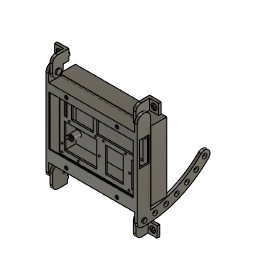
display (Autodesk Fusion 360 design; units mm, degrees)
Autodesk Fusion 360 part; units mm, degrees
note: some values were not read from the file. Set by a fixed rule: which face or edge a step refers to.
sketch "Sketch1" plane through (0, 0, 0) normal (0, 1, 0) x (1, 0, 0) in component "Frame"
  line L0 (0, 0) -> (166, 0)
  line L1 (166, 0) -> (166, -124)
  line L2 (166, -124) -> (0, -124)
  line L3 (0, -124) -> (0, 0)
  circle A0 centre (4.25, -4.25) radius 1.75
  circle A1 centre (161.75, -4.25) radius 1.75
  circle A2 centre (4.25, -119.75) radius 1.75
  circle A3 centre (161.75, -119.75) radius 1.75
  circle A4 centre (17.75, -119.75) radius 1.75
  circle A5 centre (67.45, -119.75) radius 1.75
  circle A6 centre (17.75, -60.75) radius 1.75
  circle A7 centre (67.45, -60.75) radius 1.75
  circle A8 centre (82.45, -60.75) radius 1.75
  circle A9 centre (124.45, -60.75) radius 1.75
  circle A10 centre (131.95, -32.75) radius 1.75
  circle A11 centre (74.95, -32.75) radius 1.75
  line L4 (8.5, -8.5) -> (8.5, -115.5)
  line L5 (157.5, -115.5) -> (157.5, -8.5)
  line L6 (22, -115.5) -> (22, -65)
  line L7 (22, -65) -> (63.2, -65)
  line L8 (63.2, -65) -> (63.2, -115.5)
  line L9 (69.95, -115.5) -> (69.95, -65)
  line L10 (69.95, -56.5) -> (13.5, -56.5)
  line L11 (13.5, -65) -> (13.5, -115.5)
  line L12 (69.95, -65) -> (157.5, -65)
  line L13 (69.95, -56.5) -> (69.95, -8.5)
  line L14 (86.7, -56.5) -> (86.7, -8.5)
  line L15 (120.2, -56.5) -> (120.2, -8.5)
  line L16 (136.2, -56.5) -> (136.2, -8.5)
  line L17 (86.7, -56.5) -> (120.2, -56.5)
  line L18 (136.2, -56.5) -> (157.5, -56.5)
  line L19 (69.95, -8.5) -> (8.5, -8.5)
  line L20 (157.5, -8.5) -> (136.2, -8.5)
  line L21 (120.2, -8.5) -> (86.7, -8.5)
  line L22 (8.5, -115.5) -> (13.5, -115.5)
  line L23 (22, -115.5) -> (63.2, -115.5)
  line L24 (69.95, -115.5) -> (157.5, -115.5)
  circle A12 centre (35, -119.75) radius 1.75
  circle A13 centre (131, -119.75) radius 1.75
  circle A14 centre (131, -4.25) radius 1.75
  circle A15 centre (35, -4.25) radius 1.75
  line L25 (13.5, -65) -> (8.5, -65)
  line L26 (13.5, -56.5) -> (8.5, -56.5)
  circle A16 centre (161.75, -105.5) radius 1.75
  circle A17 centre (161.75, -18.5) radius 1.75
  circle A18 centre (4.25, -18.5) radius 1.75
  circle A19 centre (4.25, -105.5) radius 1.75
  dimension "d1" = 3.5
  dimension "d2" = 2.5
  dimension "d3" = 2.5
  dimension "d4" = 112
  dimension "d5" = 154
  dimension "d6" = 2.5
  dimension "d7" = 2.5
  dimension "d8" = 10
  dimension "d9" = 46.2
  dimension "d10" = 55.5
  dimension "d11" = 7.5
  dimension "d12" = 7.5
  dimension "d13" = 38.5
  dimension "d14" = 28
  dimension "d15" = 2.5
  dimension "d16" = 2.5
  dimension "d17" = 2.5
  dimension "d18" = 2.5
  dimension "d19" = 2.5
  dimension "d20" = 2.5
  dimension "d21" = 2.5
  dimension "d22" = 2.5
  dimension "d23" = 2.5
  dimension "d24" = 2.5
  dimension "d25" = 5
  dimension "d26" = 2.5
  dimension "d27" = 2.5
  dimension "d28" = 2.5
  dimension "d29" = 35
  dimension "d30" = 35
  dimension "d44" = 10
  dimension "d45" = 10
  constraint horizontal L0
  constraint vertical L1
  constraint horizontal L2
  constraint vertical L3
  constraint coincident L0.start L3.end
  constraint equal A0 A1
  constraint equal A0 A2
  constraint equal A0 A3
  constraint vertical A0.centre A2.centre
  constraint horizontal A0.centre A1.centre
  constraint horizontal A2.centre A3.centre
  constraint vertical A1.centre A3.centre
  constraint equal A2 A4
  constraint horizontal A2.centre A4.centre
  constraint horizontal A4.centre A5.centre
  constraint equal A4 A5
  constraint horizontal A6.centre A7.centre
  constraint vertical A5.centre A7.centre
  constraint vertical A4.centre A6.centre
  constraint equal A6 A7
  constraint equal A5 A7
  constraint equal A7 A8
  constraint equal A8 A9
  constraint equal A8 A11
  constraint equal A9 A10
  constraint horizontal A7.centre A8.centre
  constraint horizontal A8.centre A9.centre
  constraint horizontal A10.centre A11.centre
  constraint perpendicular L0 L4
  constraint perpendicular L4 L22
  constraint perpendicular L5 L22
  constraint perpendicular L5 L20
  constraint coincident L6.start L22
  constraint perpendicular L6 L22
  constraint perpendicular L6 L7
  constraint coincident L8.end L22
  constraint perpendicular L8 L22
  constraint coincident L9.start L22
  constraint perpendicular L9 L22
  constraint perpendicular L9 L10
  constraint perpendicular L11 L22
  constraint coincident L5 L12.end
  constraint perpendicular L5 L12
  constraint coincident L5 L18.end
  constraint perpendicular L5 L17
  constraint collinear L7 L12
  constraint coincident L10.start L17
  constraint coincident L13.end L20
  constraint perpendicular L13 L20
  constraint perpendicular L14 L20
  constraint coincident L15.end L20
  constraint perpendicular L15 L20
  constraint coincident L16.start L17
  constraint perpendicular L16 L17
  constraint collinear L9 L13
  constraint collinear L17 L18
  constraint collinear L19 L20
  constraint collinear L20 L21
  constraint collinear L10 L17
  constraint collinear L22 L23
  constraint collinear L23 L24
  constraint horizontal A4.centre A12.centre
  constraint equal A4 A12
  constraint horizontal A3.centre A13.centre
  constraint equal A3 A13
  constraint horizontal A14.centre A15.centre
  constraint equal A0 A15
  constraint equal A14 A15
  constraint vertical A12.centre A15.centre
  constraint vertical A13.centre A14.centre
  constraint horizontal A0.centre A15.centre
  constraint coincident L4 L25.end
  constraint perpendicular L4 L25
  constraint coincident L4 L26.end
  constraint perpendicular L4 L26
  constraint collinear L7 L25
  constraint equal A16 A17
  constraint equal A17 A18
  constraint equal A18 A19
  constraint equal A1 A17
  constraint vertical A16.centre A17.centre
  constraint vertical A1.centre A17.centre
  constraint vertical A0.centre A18.centre
  constraint vertical A18.centre A19.centre
  constraint horizontal A16.centre A19.centre
  constraint horizontal A17.centre A18.centre
  measures "d1" diameter of A0
  measures "d2" distance of L3 A0
  measures "d3" distance of L0 A0
  measures "d4" distance of A0 A2
  measures "d5" distance of A0 A1
  measures "d6" distance of L1 A1
  measures "d7" distance of L2 A2
  measures "d8" distance of A2 A4
  measures "d9" distance of A4 A5
  measures "d10" distance of A4 A6
  measures "d11" horizontal distance of A8.centre A11.centre
  measures "d12" horizontal distance of A9.centre A10.centre
  measures "d13" distance of A8 A9
  measures "d14" vertical distance of A8.centre A11.centre
  measures "d15" distance of A0 L4
  measures "d16" distance of A0 L20
  measures "d17" distance of A2 L22
  measures "d18" distance of A1 L5
  measures "d19" distance of A4 L6
  measures "d20" distance of A4 L11
  measures "d21" distance of A6 L7
  measures "d22" distance of A6 L10
  measures "d23" distance of A5 L8
  measures "d24" distance of A5.centre L9
  measures "d25" distance of A11.centre L13
  measures "d26" distance of A8 L14
  measures "d27" distance of A9 L15
  measures "d28" distance of A10 L16
  measures "d29" distance of L3 A12.centre
  measures "d30" distance of L1 A13.centre
  measures "d44" distance of L20 A17.centre
  measures "d45" distance of L24 A16.centre
extrude "Extrude1" add sketch "Sketch1" along normal blind 3 makes body 1 in component "Frame"
sketch "Sketch4" plane through (0, 0, 0) normal (0, 0, -1) x (1, 0, 0) in component "Frame"
  line L0 (166, 0) -> (0, 0)
  line L1 (0, 0) -> (0, -3)
  line L2 (0, -3) -> (166, -3)
  line L3 (166, -3) -> (166, 0)
  line L4 (157, -3) -> (142, -3)
  line L5 (142, -3) -> (142, -9.5)
  line L6 (157, -9.5) -> (157, -3)
  arc A0 (142, -9.5) -> (157, -9.5) centre (149.5, -9.5) ccw
  circle A1 centre (149.5, -9.5) radius 3.75
  circle A2 centre (149.5, -9.5) radius 5.5
  line L7 (142, -3) -> (136, -3)
  line L8 (136, -3) -> (136, -12.5)
  line L9 (136, -12.5) -> (142, -12.5)
  line L10 (142, -9.5) -> (142, -3)
  line L11 (140.5, -5) -> (137.5, -5)
  line L12 (137.5, -5) -> (137.5, -10.5)
  line L13 (137.5, -10.5) -> (140.5, -10.5)
  line L14 (140.5, -10.5) -> (140.5, -5)
  line L15 (142, -12.5) -> (142.6261, -12.5)
  point P0 (157.5, -3)
  dimension "d34" = 15
  dimension "d35" = 6.5
  dimension "d37" = 0.5
  dimension "d38" = 7.5
  dimension "d39" = 11
  dimension "d46" = 3
  dimension "d47" = 1.5
  dimension "d48" = 1.5
  dimension "d49" = 5.5
  dimension "d50" = 2
  dimension "d51" = 2
  constraint horizontal L4
  constraint vertical L5
  constraint vertical L6
  constraint coincident L2 L4.start
  constraint tangent L5 A0
  constraint equal L5 L6
  constraint concentric A0 A1
  constraint concentric A1 A2
  constraint horizontal L7
  constraint vertical L8
  constraint horizontal L9
  constraint vertical L10
  constraint horizontal L11
  constraint vertical L12
  constraint horizontal L13
  constraint vertical L14
  constraint coincident A0 L15.end
  constraint perpendicular L10 L15
  measures "d34" distance of L5.end L6.start
  measures "d35" distance of L4.start L6.start
  measures "d37" distance of L6 P0
  measures "d38" diameter of A1
  measures "d39" diameter of A2
  measures "d46" distance of L12.end L13.end
  measures "d47" distance of L10 L14
  measures "d48" distance of L8 L12
  measures "d49" distance of L11.end L12.end
  measures "d50" distance of L7 L11
  measures "d51" distance of L9 L13
extrude "Extrude2" add sketch "Sketch4" against normal blind 2.5 separate body contours A2 makes body 2 in component "Frame"
extrude "Extrude3" add sketch "Sketch4" against normal up to surface (8.5 mm away) contours L2 L4 L5 L6 A0 L10 bodies 1 2 in component "Frame"
extrude "Extrude4" add sketch "Sketch4" against normal up to surface (8.5 mm away) contours L2 L5 A0 L7 L8 L9 L10 L15 bodies 1 in component "Frame"
ref_plane "WorkPlane1" through (83, 15, 62) normal (0, 1, 0) x (1, 0, 0) in component "Abdeckung Hinten"
sketch "Sketch1 (2)" plane through (83, 15, 62) normal (0, 1, 0) x (1, 0, 0) in component "Abdeckung Hinten"
  circle A0 centre (78.75, 43.5) radius 1.75
  circle A1 centre (78.75, -43.5) radius 1.75
  circle A2 centre (-78.75, -43.5) radius 1.75
  circle A3 centre (-78.75, 43.5) radius 1.75
  circle A4 centre (-78.75, -43.5) radius 1.75
  circle A5 centre (-78.75, 43.5) radius 1.75
  circle A6 centre (78.75, 43.5) radius 1.75
  circle A7 centre (78.75, -43.5) radius 1.75
  circle A8 centre (78.75, -43.5) radius 3.75
  circle A9 centre (78.75, 43.5) radius 3.75
  circle A10 centre (-78.75, -43.5) radius 3.75
  circle A11 centre (-78.75, 43.5) radius 3.75
  dimension "d56" = 2
  dimension "d57" = 2
  dimension "d58" = 2
  dimension "d59" = 2
  constraint equal A2 A4
  constraint equal A3 A5
  constraint equal A0 A6
  constraint equal A1 A7
  constraint concentric A1 A7
  constraint concentric A0 A6
  constraint concentric A2 A4
  constraint concentric A3 A5
extrude "Extrude1'" add sketch "Sketch1 (2)" along normal blind 2 separate body makes body 3 at (162.7657, 16.3333, 14.8902) makes body 4 at (7.9814, 15.6667, 18.8734) makes body 5 at (162.7657, 16.3333, 101.8902) makes body 6 at (7.884, 16.3333, 104.5747) in component "Abdeckung Hinten"
sketch "Sketch4 (2)" plane through (0, 17, 0) normal (0, 1, 0) x (-1, 0, 0) in component "Abdeckung Hinten"
  circle A0 centre (-4.25, 105.5) radius 1.75
  circle A1 centre (-4.25, 105.5) radius 3.75 construction
  circle A2 centre (-4.25, 105.5) radius 5.75
  circle A3 centre (-4.25, 18.5) radius 5.75
  circle A4 centre (-4.25, 18.5) radius 3.75 construction
  circle A5 centre (-161.75, 18.5) radius 5.75
  circle A6 centre (-161.75, 105.5) radius 5.75
  circle A7 centre (-161.75, 18.5) radius 3.75 construction
  circle A8 centre (-161.75, 105.5) radius 3.75 construction
  circle A9 centre (-4.25, 18.5) radius 1.75
  circle A10 centre (-4.25, 18.5) radius 1.75
  circle A11 centre (-161.75, 18.5) radius 1.75
  circle A12 centre (-161.75, 18.5) radius 1.75
  circle A13 centre (-161.75, 105.5) radius 1.75
  circle A14 centre (-161.75, 105.5) radius 1.75
  dimension "d65" = 2
  constraint concentric A3 A4
  constraint equal A2 A3
  constraint equal A5 A6
  constraint equal A3 A5
  constraint concentric A5 A7
  constraint concentric A6 A8
  constraint concentric A9 A10
  constraint equal A9 A10
  constraint equal A11 A12
  constraint concentric A11 A12
  constraint equal A13 A14
  constraint concentric A13 A14
extrude "Extrude2'" add sketch "Sketch4 (2)" along normal blind 2 bodies 3 4 5 6 in component "Abdeckung Hinten"
sketch "Sketch5" plane through (0, 19, 0) normal (0, 1, 0) x (-1, 0, 0) in component "Abdeckung Hinten"
  circle A0 centre (-4.25, 105.5) radius 1.75
  circle A1 centre (-4.25, 105.5) radius 5.75
  circle A2 centre (-4.25, 105.5) radius 3.35
  circle A3 centre (-4.25, 18.5) radius 3.35
  circle A4 centre (-161.75, 18.5) radius 3.35
  circle A5 centre (-161.75, 105.5) radius 3.35
  circle A6 centre (-161.75, 18.5) radius 1.75
  circle A7 centre (-161.75, 105.5) radius 1.75
  circle A8 centre (-4.25, 18.5) radius 1.75
  circle A9 centre (-161.75, 105.5) radius 5.75
  circle A10 centre (-161.75, 18.5) radius 5.75
  circle A11 centre (-4.25, 18.5) radius 5.75
  circle A12 centre (-4.25, 105.5) radius 5.75
  circle A13 centre (-4.25, 18.5) radius 5.75
  circle A14 centre (-161.75, 18.5) radius 5.75
  circle A15 centre (-161.75, 105.5) radius 5.75
  dimension "d68" = 1.6
  dimension "d69" = 1.4
  constraint equal A2 A3
  constraint equal A3 A4
  constraint equal A4 A5
  constraint concentric A4 A6
  constraint concentric A5 A7
  constraint concentric A3 A8
  constraint concentric A7 A9
  constraint concentric A4 A10
  constraint concentric A8 A11
  constraint concentric A0 A12
  constraint equal A1 A12
  constraint equal A11 A13
  constraint equal A10 A14
  constraint equal A9 A15
extrude "Extrude3'" add sketch "Sketch5" along normal blind 12 contours A1 A12 | A9 A15 | A10 A14 | A11 A13 bodies 3 4 5 6 in component "Abdeckung Hinten"
ref_plane "WorkPlane2" through (161.75, 31, 105.5) normal (0, 1, 0) x (-1, 0, 0) in component "Abdeckung Hinten"
sketch "Sketch8" plane through (161.75, 31, 105.5) normal (0, 1, 0) x (1, 0, 0) in component "Abdeckung Hinten"
  line L0 (7.75, -22) -> (-165.25, -22)
  line L1 (-165.25, -22) -> (-165.25, 109)
  line L2 (-165.25, 109) -> (7.75, 109)
  line L3 (7.75, 109) -> (7.75, -22)
  line L4 (4.25, 105.5) -> (4.25, -18.5)
  line L5 (4.25, -18.5) -> (-161.75, -18.5)
  line L6 (-161.75, 105.5) -> (4.25, 105.5)
  line L7 (-161.75, -18.5) -> (-161.75, 105.5)
  circle A0 centre (-157.5, 0) radius 3.35
  circle A1 centre (-157.5, 0) radius 3.35
  circle A2 centre (-157.5, 87) radius 3.35
  circle A3 centre (-157.5, 87) radius 3.35
  circle A4 centre (0, 87) radius 3.35
  circle A5 centre (0, 87) radius 3.35
  circle A6 centre (0, 0) radius 3.35
  circle A7 centre (0, 0) radius 3.35
  dimension "d81" = 3.5
  dimension "d82" = 3.5
  dimension "d83" = 3.5
  dimension "d84" = 3.5
  constraint horizontal L0
  constraint vertical L1
  constraint horizontal L2
  constraint vertical L3
  constraint equal A0 A1
  constraint concentric A0 A1
  constraint equal A2 A3
  constraint concentric A2 A3
  constraint equal A4 A5
  constraint concentric A4 A5
  constraint equal A6 A7
  constraint concentric A6 A7
  measures "d81" distance of L3 L4
  measures "d82" distance of L0 L5
  measures "d83" distance of L2 L6
  measures "d84" distance of L1 L7
extrude "Extrude4'" add sketch "Sketch8" along normal blind 2 contours L0 L1 L2 L3 | L4 L5 L6 L7 bodies 3 4 5 6 in component "Abdeckung Hinten"
sketch "Sketch9" plane through (0, 31, 0) normal (0, -1, 0) x (1, 0, 0) in component "Abdeckung Hinten"
  circle A0 centre (4.25, 105.5) radius 5.75
  circle A1 centre (161.75, 105.5) radius 5.75
  circle A2 centre (4.25, 18.5) radius 5.75
  line L0 (-3.5, -3.5) -> (169.5, -3.5)
  line L1 (169.5, -3.5) -> (169.5, 127.5)
  line L2 (169.5, 127.5) -> (-3.5, 127.5)
  line L3 (-3.5, 127.5) -> (-3.5, -3.5)
  circle A3 centre (161.75, 18.5) radius 5.75
  line L4 (-0.5, -0.5) -> (166.5, -0.5)
  line L5 (166.5, -0.5) -> (166.5, 124.5)
  line L6 (166.5, 124.5) -> (-0.5, 124.5)
  line L7 (-0.5, 124.5) -> (-0.5, -0.5)
  dimension "d87" = -3
extrude "Extrude5" add sketch "Sketch9" along normal up to surface (31 mm away) bodies 3 in component "Abdeckung Hinten"
sketch "Sketch10" plane through (0, 0, 0) normal (0, -1, 0) x (1, 0, 0) in component "Abdeckung Hinten"
  arc A0 (-0.5, 108.7404) -> (-0.5, 102.2596) centre (4.25, 105.5) ccw
  line L0 (-0.5, 108.7404) -> (-0.5, 124.5)
  line L1 (-0.5, 124.5) -> (166.5, 124.5)
  line L2 (166.5, 124.5) -> (166.5, 108.7404)
  arc A1 (166.5, 102.2596) -> (166.5, 108.7404) centre (161.75, 105.5) ccw
  line L3 (166.5, 102.2596) -> (166.5, 21.7404)
  arc A2 (166.5, 15.2596) -> (166.5, 21.7404) centre (161.75, 18.5) ccw
  line L4 (166.5, 15.2596) -> (166.5, -0.5)
  line L5 (166.5, -0.5) -> (-0.5, -0.5)
  line L6 (-0.5, -0.5) -> (-0.5, 15.2596)
  arc A3 (-0.5, 21.7404) -> (-0.5, 15.2596) centre (4.25, 18.5) ccw
  line L7 (-0.5, 21.7404) -> (-0.5, 102.2596)
  line L8 (169.5, 127.5) -> (-3.5, 127.5)
  line L9 (-3.5, 127.5) -> (-3.5, -3.5)
  line L10 (-3.5, -3.5) -> (169.5, -3.5)
  line L11 (169.5, -3.5) -> (169.5, 127.5)
  line L12 (-1.9, -1.9) -> (167.9, -1.9)
  line L13 (167.9, -1.9) -> (167.9, 125.9)
  line L14 (167.9, 125.9) -> (-1.9, 125.9)
  line L15 (-1.9, 125.9) -> (-1.9, -1.9)
  dimension "d90" = -1.6
extrude "Extrude6" cut sketch "Sketch10" against normal blind 3 contours L8 L9 L10 L11 bodies 3 in component "Abdeckung Hinten"
sketch "Sketch11" plane through (0, 0, -0.5) normal (0, 0, 1) x (-1, 0, 0) in component "Abdeckung Hinten"
  line L0 (0.5, 0) -> (-166.5, 0)
  line L1 (-166.5, 0) -> (-166.5, -31)
  line L2 (-166.5, -31) -> (0.5, -31)
  line L3 (0.5, -31) -> (0.5, 0)
  line L4 (-157, -3) -> (-136, -3) construction
  line L5 (-157, -9.5) -> (-157, -3) construction
  line L6 (0, -3) -> (-166, -3)
  line L7 (-157, -9.5) -> (-157, -3)
  line L8 (-136, -3) -> (-136, -12.5) construction
  line L9 (-136, -3) -> (-136, -12.5)
  arc A0 (-157, -9.5) -> (-142.6261, -12.5) centre (-149.5, -9.5) ccw
  arc A1 (-157, -9.5) -> (-142.6261, -12.5) centre (-149.5, -9.5) ccw construction
  line L10 (-142.6261, -12.5) -> (-136, -12.5) construction
  line L11 (-137, -4) -> (-137, -11.5)
  line L12 (-143.3153, -11.5) -> (-137, -11.5)
  arc A2 (-156, -9.5) -> (-143.3153, -11.5) centre (-149.5, -9.5) ccw
  line L13 (-156, -9.5) -> (-156, -4)
  line L14 (-156, -4) -> (-137, -4)
  dimension "d93" = -1
  constraint horizontal L4
  constraint vertical L5
  constraint collinear L4 L6
  constraint collinear L5 L7
  constraint perpendicular L6 L8
  constraint equal L8 L9
  constraint collinear L8 L9
  constraint equal A0 A1
  constraint concentric A0 A1
  constraint coincident A0.end A1.end
extrude "Extrude7" cut sketch "Sketch11" against normal up to surface (3 mm away) contours L11 L12 A2 L13 L14 bodies 3 in component "Abdeckung Hinten"
ref_plane "WorkPlane1" through (83, -12, 62) normal (0, -1, 0) x (-1, 0, 0) in component "Display Halterung"
sketch "Sketch1 (3)" plane through (83, -12, 62) normal (0, -1, 0) x (1, 0, 0) in component "Display Halterung"
  circle A0 centre (-48, 57.75) radius 1.75
  circle A1 centre (48, 57.75) radius 1.75
  circle A2 centre (-48, -57.75) radius 1.75
  circle A3 centre (48, -57.75) radius 1.75
  circle A4 centre (-48, 57.75) radius 1.75
  circle A5 centre (48, 57.75) radius 1.75
  circle A6 centre (48, -57.75) radius 1.75
  circle A7 centre (-48, -57.75) radius 1.75
  circle A8 centre (-48, 57.75) radius 3.75
  circle A9 centre (48, 57.75) radius 3.75
  circle A10 centre (48, -57.75) radius 3.75
  circle A11 centre (-48, -57.75) radius 3.75
  dimension "d97" = 2
  dimension "d98" = 2
  dimension "d99" = 2
  dimension "d100" = 2
  constraint equal A0 A4
  constraint equal A1 A5
  constraint equal A3 A6
  constraint equal A2 A7
  constraint concentric A2 A7
  constraint concentric A3 A6
  constraint concentric A1 A5
  constraint concentric A0 A4
extrude "Extrude1''" add sketch "Sketch1 (3)" along normal blind 6.5 separate body makes body 7 at (132.0157, -16.3333, 7.8598) makes body 8 at (132.0157, -16.3333, 123.3598) makes body 9 at (38.7314, -14.1667, 3.8766) makes body 10 at (38.634, -16.3333, 120.6753) in component "Display Halterung"
ref_plane "WorkPlane2" through (83, -18.5, 62) normal (0, -1, 0) x (-1, 0, 0) in component "Display Halterung"
sketch "Sketch2" plane through (83, -18.5, 62) normal (0, -1, 0) x (1, 0, 0) in component "Display Halterung"
  line L0 (-86.5, 65.5) -> (86.5, 65.5)
  line L1 (86.5, 65.5) -> (86.5, -65.5)
  line L2 (86.5, -65.5) -> (-86.5, -65.5)
  line L3 (-86.5, -65.5) -> (-86.5, 65.5)
  line L4 (-86.5, 65.5) -> (86.5, 65.5)
  line L5 (86.5, 65.5) -> (86.5, -65.5)
  line L6 (86.5, -65.5) -> (-86.5, -65.5)
  line L7 (-86.5, -65.5) -> (-86.5, 65.5)
  line L8 (-83, 53.5) -> (83, 53.5)
  line L9 (83, 53.5) -> (83, -47.6)
  line L10 (83, -47.6) -> (-83, -47.6)
  line L11 (-83, -47.6) -> (-83, 53.5)
  line L12 (-83, 62) -> (-83, -62)
  line L13 (83, -62) -> (83, 62)
  line L14 (74.5, 53.5) -> (-13.05, 53.5)
  circle A0 centre (48, -57.75) radius 1.75
  circle A1 centre (-48, 57.75) radius 1.75
  circle A2 centre (48, 57.75) radius 1.75
  circle A3 centre (-48, -57.75) radius 1.75
  dimension "d105" = 166
  dimension "d106" = 100.8
  dimension "d107" = 8.4
  dimension "d108" = 3.5
  dimension "d109" = 3.5
  dimension "d110" = 3.5
  constraint horizontal L0
  constraint vertical L1
  constraint horizontal L2
  constraint vertical L3
  constraint collinear L0 L4
  constraint collinear L1 L5
  constraint collinear L2 L6
  constraint collinear L3 L7
  constraint horizontal L8
  constraint vertical L9
  constraint horizontal L10
  constraint vertical L11
  constraint collinear L11 L12
  constraint collinear L9 L13
  constraint collinear L8 L14
  measures "d105" distance of L8.start L8.end
  measures "d107" distance of L10 A0
  measures "d108" diameter of A1
  measures "d109" diameter of A2
  measures "d110" diameter of A3
extrude "Extrude2''" add sketch "Sketch2" along normal blind 2.8 bodies 7 8 9 10 in component "Display Halterung"
sketch "Sketch3" plane through (0, -21.3, 0) normal (0, -1, 0) x (1, 0, 0) in component "Display Halterung"
  circle A0 centre (131, 119.75) radius 1.75
  circle A1 centre (35, 119.75) radius 1.75
  circle A2 centre (131, 4.25) radius 1.75
  line L0 (166, 115.5) -> (166, 14.4) construction
  line L1 (166, 14.4) -> (0, 14.4) construction
  line L2 (0, 14.4) -> (0, 115.5) construction
  line L3 (0, 115.5) -> (166, 115.5) construction
  circle A3 centre (35, 4.25) radius 1.75
  line L4 (-3.5, -3.5) -> (169.5, -3.5)
  line L5 (169.5, -3.5) -> (169.5, 127.5)
  line L6 (169.5, 127.5) -> (-3.5, 127.5)
  line L7 (-3.5, 127.5) -> (-3.5, -3.5)
  line L8 (2, 112.5) -> (162, 112.5)
  line L9 (162, 112.5) -> (162, 18.9)
  line L10 (162, 18.9) -> (2, 18.9)
  line L11 (2, 18.9) -> (2, 112.5)
  dimension "d113" = 4
  dimension "d114" = 3
  dimension "d115" = 2
  dimension "d116" = 4.5
  constraint horizontal L8
  constraint vertical L9
  constraint horizontal L10
  constraint vertical L11
  measures "d113" distance of L0 L9
  measures "d114" distance of L3 L8
  measures "d115" distance of L2 L11
  measures "d116" distance of L1 L10
extrude "Extrude3''" add sketch "Sketch3" along normal blind 1.5 bodies 7 in component "Display Halterung"
sketch "Sketch4 (3)" plane through (0, -22.8, 0) normal (0, -1, 0) x (1, 0, 0) in component "Display Halterung"
  circle A0 centre (35, 119.75) radius 1.75
  circle A1 centre (131, 4.25) radius 1.75
  circle A2 centre (35, 4.25) radius 1.75
  circle A3 centre (131, 119.75) radius 1.75
  line L0 (162, 18.9) -> (2, 18.9)
  line L1 (2, 18.9) -> (2, 112.5)
  line L2 (2, 112.5) -> (162, 112.5)
  line L3 (162, 112.5) -> (162, 18.9)
  line L4 (-3.5, 127.5) -> (-3.5, -3.5)
  line L5 (-3.5, -3.5) -> (169.5, -3.5)
  line L6 (169.5, -3.5) -> (169.5, 127.5)
  line L7 (169.5, 127.5) -> (-3.5, 127.5)
  circle A4 centre (131, 119.75) radius 3.25
  circle A5 centre (35, 119.75) radius 3.25
  circle A6 centre (131, 4.25) radius 3.25
  circle A7 centre (35, 4.25) radius 3.25
  dimension "d119" = 1.5
  dimension "d120" = 1.5
  dimension "d121" = 1.5
  dimension "d122" = 1.5
extrude "Extrude4''" cut sketch "Sketch4 (3)" against normal blind 2 contours A4 | A5 | A6 | A7 bodies 7 in component "Display Halterung"
sketch "Sketch5 (2)" plane through (0, -18.5, 0) normal (0, 1, 0) x (-1, 0, 0) in component "Display Halterung"
  circle A0 centre (-35, 119.75) radius 3.75
  circle A1 centre (-35, 4.25) radius 3.75
  circle A2 centre (-131, 119.75) radius 3.75
  line L0 (-169.5, -3.5) -> (3.5, -3.5)
  line L1 (3.5, -3.5) -> (3.5, 127.5)
  line L2 (3.5, 127.5) -> (-169.5, 127.5)
  line L3 (-169.5, 127.5) -> (-169.5, -3.5)
  line L4 (-166, 14.4) -> (-166, 115.5)
  line L5 (-166, 115.5) -> (0, 115.5)
  line L6 (0, 115.5) -> (0, 14.4)
  line L7 (0, 14.4) -> (-166, 14.4)
  circle A3 centre (-131, 4.25) radius 3.75
  line L8 (-166.5, 124.5) -> (0.5, 124.5)
  line L9 (0.5, 124.5) -> (0.5, -0.5)
  line L10 (0.5, -0.5) -> (-166.5, -0.5)
  line L11 (-166.5, -0.5) -> (-166.5, 124.5)
  line L12 (0.5, 124.5) -> (0.5, -0.5)
  line L13 (-166.5, 124.5) -> (0.5, 124.5)
  line L14 (-166.5, -0.5) -> (-166.5, 124.5)
  line L15 (0.5, -0.5) -> (-166.5, -0.5)
  constraint horizontal L8
  constraint vertical L9
  constraint horizontal L10
  constraint vertical L11
  constraint collinear L9 L12
  constraint collinear L8 L13
  constraint collinear L11 L14
  constraint collinear L10 L15
extrude "Extrude5'" add sketch "Sketch5 (2)" along normal up to surface (18.2 mm away) contours L0 L1 L2 L3 bodies 7 in component "Display Halterung"
sketch "Sketch6" plane through (0, -0.3, 0) normal (0, 1, 0) x (-1, 0, 0) in component "Display Halterung"
  line L0 (-166.5, 124.5) -> (0.5, 124.5)
  line L1 (0.5, 124.5) -> (0.5, -0.5)
  line L2 (0.5, -0.5) -> (-166.5, -0.5)
  line L3 (-166.5, -0.5) -> (-166.5, 124.5)
  line L4 (3.5, 127.5) -> (-169.5, 127.5)
  line L5 (-169.5, 127.5) -> (-169.5, -3.5)
  line L6 (-169.5, -3.5) -> (3.5, -3.5)
  line L7 (3.5, -3.5) -> (3.5, 127.5)
  line L8 (-168.2, 126.2) -> (2.2, 126.2)
  line L9 (2.2, 126.2) -> (2.2, -2.2)
  line L10 (2.2, -2.2) -> (-168.2, -2.2)
  line L11 (-168.2, -2.2) -> (-168.2, 126.2)
  line L12 (1.9, 125.9) -> (1.9, -1.9)
  line L13 (-167.9, 125.9) -> (1.9, 125.9)
  line L14 (-167.9, -1.9) -> (-167.9, 125.9)
  line L15 (1.9, -1.9) -> (-167.9, -1.9)
  dimension "d127" = 0.3
  dimension "d128" = 0.3
  dimension "d129" = 0.3
  dimension "d130" = 0.3
  constraint horizontal L8
  constraint vertical L9
  constraint horizontal L10
  constraint vertical L11
  measures "d127" distance of L9 L12
  measures "d128" distance of L8 L13
  measures "d129" distance of L11 L14
  measures "d130" distance of L10 L15
extrude "Extrude6'" add sketch "Sketch6" along normal up to surface (2.8 mm away) contours L4 L5 L6 L7 bodies 7 in component "Display Halterung"
sketch "Sketch7" plane through (166.5, 0, 0) normal (-1, 0, 0) x (0, -1, 0) in component "Display Halterung"
  line L0 (0.3, 124.5) -> (0.3, -0.5)
  line L1 (0.3, -0.5) -> (18.5, -0.5)
  line L2 (18.5, -0.5) -> (18.5, 124.5)
  line L3 (18.5, 124.5) -> (0.3, 124.5)
  line L4 (0.3, 115) -> (19.3, 115)
  line L5 (19.3, 115) -> (19.3, 68)
  line L6 (19.3, 68) -> (0.3, 68)
  line L7 (0.3, 68) -> (0.3, 115)
  line L8 (0, 124) -> (-3, 124)
  dimension "d133" = 19
  dimension "d134" = 9
  dimension "d135" = 47
  constraint horizontal L4
  constraint vertical L5
  constraint horizontal L6
  constraint vertical L7
  constraint coincident L0 L4.start
  measures "d133" distance of L4.start L4.end
  measures "d134" distance of L4 L8
  measures "d135" distance of L4.start L6.end
extrude "Extrude7'" cut sketch "Sketch7" against normal up to surface (3 mm away) contours L0 L2 L4 L6 L7 bodies 7 in component "Display Halterung"
sketch "Sketch9 (2)" plane through (-3.5, 0, 0) normal (-1, 0, 0) x (0, -1, 0) in component "Display Halterung"
  line L0 (-2.5, -3.5) -> (22.8, -3.5)
  line L1 (22.8, -3.5) -> (22.8, 127.5)
  line L2 (22.8, 127.5) -> (-2.5, 127.5)
  line L3 (-2.5, 127.5) -> (-2.5, -3.5)
  line L4 (-2.5, 127.5) -> (22.8, 127.5)
  line L5 (22.8, 127.5) -> (22.8, 142.5)
  line L6 (-2.5, 142.5) -> (-2.5, 127.5)
  arc A0 (22.8, 142.5) -> (-2.5, 142.5) centre (10.15, 142.5) ccw
  dimension "d140" = 15
  dimension "d141" = 25.3
  constraint horizontal L4
  constraint vertical L5
  constraint vertical L6
  constraint coincident L2.end L3.start
  constraint tangent L5 A0
  constraint collinear L1 L5
  constraint tangent L6 A0
  measures "d140" distance of L2.end L6.start
  measures "d141" distance of L5.end L6.start
extrude "Extrude8" add sketch "Sketch9 (2)" against normal blind 5 contours L2 L4 L5 L6 A0 bodies 7 in component "Display Halterung"
extrude "Extrude9" add sketch "Sketch9 (2)" along normal blind 5 from surface at -173 contours L2 L4 L5 L6 A0 bodies 7 in component "Display Halterung"
sketch "Sketch10 (2)" plane through (1.5, 0, 0) normal (1, 0, 0) x (0, 1, 0) in component "Display Halterung"
  arc A0 (2.5, 142.5) -> (-22.8, 142.5) centre (-10.15, 142.5) ccw
  line L0 (-22.8, 142.5) -> (-22.8, 127.5)
  line L1 (-22.8, 127.5) -> (2.5, 127.5)
  line L2 (2.5, 127.5) -> (2.5, 142.5)
  circle A1 centre (-10.15, 142.5) radius 5
  dimension "d147" = 10
  constraint concentric A0 A1
  measures "d147" diameter of A1
extrude "Extrude10" add sketch "Sketch10 (2)" along normal blind 7 contours A1 bodies 7 in component "Display Halterung"
extrude "Extrude11" add sketch "Sketch10 (2)" against normal blind 7 from surface at 163 contours A1 bodies 7 in component "Display Halterung"
sketch "Sketch11 (2)" plane through (-3.5, 0, 0) normal (-1, 0, 0) x (0, -1, 0) in component "Display Halterung"
  circle A0 centre (10.15, 142.5) radius 5
  arc A1 (-98.0373, 34.3127) -> (10.15, -10.5) centre (10.15, 142.5) ccw
  line L0 (10.15, 142.5) -> (-98.0373, 34.3127) construction
  line L1 (10.15, 142.5) -> (10.15, -10.5) construction
  arc A2 (-112.1795, 20.1705) -> (10.15, -30.5) centre (10.15, 142.5) ccw
  line L2 (22.8, -3.5) -> (-2.5, -3.5)
  line L3 (-2.5, -3.5) -> (-2.5, -9.9762)
  line L4 (22.8, -20.5) -> (22.8, -3.5)
  line L5 (-2.5, -3.5) -> (22.8, -3.5)
  line L6 (-2.5, 142.5) -> (-2.5, -3.5)
  line L7 (22.8, -3.5) -> (22.8, 142.5)
  line L8 (10.15, -30.5) -> (12.8, -30.5)
  arc A3 (-98.0373, 34.3127) -> (-112.1795, 20.1705) centre (-105.1084, 27.2416) ccw
  circle A4 centre (10.15, -20.5) radius 4.4
  circle A5 centre (-11.1258, -19.1055) radius 4.4
  circle A6 centre (-32.0375, -14.9459) radius 4.4
  circle A7 centre (-52.2274, -8.0924) radius 4.4
  circle A8 centre (-71.35, 1.3379) radius 4.4
  circle A9 centre (-89.0781, 13.1834) radius 4.4
  circle A10 centre (-105.1084, 27.2416) radius 4.4
  arc A11 (12.8, -30.5) -> (22.8, -20.5) centre (12.8, -20.5) ccw
  point P0 (22.8, -30.5)
  dimension "d182" = 45
  dimension "d183" = 20
  dimension "d184" = 27
  dimension "d199" = 8.8
  dimension "d200" = 12.65
  dimension "d201" = 25.3
  dimension "d202" = 10
  dimension "d204" = -45
  dimension "d205" = 10
  constraint coincident A0.centre A1.centre
  constraint horizontal L2
  constraint vertical L3
  constraint vertical L4
  constraint collinear L2 L5
  constraint collinear L3 L6
  constraint collinear L4 L7
  constraint perpendicular L4 L8
  constraint tangent A2 L8
  constraint coincident A1 L3.end
  constraint tangent A1 A3
  constraint coincident P0 L4
  constraint coincident P0 L8
  constraint tangent L4 A11
  constraint tangent L8 A11
  measures "d182" angle of L0 L1
  measures "d184" distance of L2.start P0
  measures "d199" diameter of A4
  measures "d200" distance of L4 A4.centre
  measures "d201" distance of L2.start L2.end
  measures "d202" distance of L8 A4.centre
  measures "d205" radius of A11
extrude "Extrude18" add sketch "Sketch11 (2)" against normal up to surface (5 mm away) contours A1 A2 L2 L3 L4 L5 L8 A3 A11 bodies 7 in component "Display Halterung"
extrude "Extrude19" add sketch "Sketch11 (2)" along normal up to surface (5 mm away) from surface at -173 contours A1 A2 L2 L3 L4 L5 L8 A3 A11 bodies 7 in component "Display Halterung"
sketch "Sketch1 (4)" plane through (1.5, 0, 0) normal (1, 0, 0) x (0, 1, 0) in component "Geruesthalterung Top"
  circle A0 centre (-10.15, 142.5) radius 5
  arc A1 (2.5, 142.5) -> (-22.8, 142.5) centre (-10.15, 142.5) ccw construction
  line L0 (-22.8, 142.5) -> (-22.8, 127.5)
  line L1 (-22.8, 127.5) -> (2.5, 127.5)
  line L2 (2.5, 127.5) -> (2.5, 142.5)
  circle A2 centre (-10.15, 142.5) radius 5.25
  line L3 (-0.15, 142.5) -> (-0.15, 149.5)
  line L4 (10.5, 169.5) -> (-10.15, 169.5)
  line L5 (-20.15, 159.5) -> (-20.15, 142.5)
  arc A3 (-20.15, 142.5) -> (-0.15, 142.5) centre (-10.15, 142.5) ccw
  arc A4 (-10.15, 169.5) -> (-20.15, 159.5) centre (-10.15, 159.5) ccw
  line L6 (10.5, 169.5) -> (10.5, 149.5)
  line L7 (10.5, 149.5) -> (-0.15, 149.5)
  dimension "d206" = 10.5
  dimension "d208" = 20
  dimension "d230" = 10
  dimension "d273" = 8
  dimension "d274" = 20
  dimension "d275" = 7
  constraint concentric A0 A2
  constraint concentric A0 A3
  constraint vertical L3
  constraint vertical L5
  constraint tangent L5 A3
  constraint tangent L3 A3
  constraint vertical L6
  constraint horizontal L7
  constraint tangent L5 A4
  constraint tangent L4 A4
  constraint horizontal L4
  measures "d206" diameter of A2
  measures "d208" diameter of A3
  measures "d230" radius of A4
  measures "d273" distance of L2 L6
  measures "d274" distance of L4.start L6.end
  measures "d275" distance of L3.start L3.end
extrude "Extrude1'''" add sketch "Sketch1 (4)" along normal blind 5 separate body contours L3 L4 L5 A3 A4 L6 L7 makes body 11 in component "Geruesthalterung Top"
sketch "Sketch2 (2)" plane through (1.5, 0, 0) normal (-1, 0, 0) x (0, -1, 0) in component "Geruesthalterung Top"
  circle A0 centre (10.15, 142.5) radius 5.25
  arc A1 (0.15, 142.5) -> (20.15, 142.5) centre (10.15, 142.5) ccw
  line L0 (20.15, 142.5) -> (20.15, 159.5)
  line L1 (10.15, 169.5) -> (-10.5, 169.5)
  line L2 (0.15, 149.5) -> (0.15, 142.5)
  line L3 (-10.5, 169.5) -> (-5.5, 169.5)
  line L4 (-5.5, 169.5) -> (-5.5, 149.5)
  line L5 (-5.5, 149.5) -> (-10.5, 149.5)
  line L6 (-10.5, 149.5) -> (-10.5, 169.5)
  arc A2 (20.15, 159.5) -> (10.15, 169.5) centre (10.15, 159.5) ccw
  line L7 (-10.5, 169.5) -> (-10.5, 149.5)
  line L8 (-10.5, 149.5) -> (0.15, 149.5)
  dimension "d212" = 20
  dimension "d213" = 5
  constraint horizontal L3
  constraint vertical L4
  constraint horizontal L5
  constraint vertical L6
  constraint coincident L1.end L3.start
  measures "d212" distance of L1.end L5.end
  measures "d213" distance of L1.end L3.end
extrude "Extrude2'''" add sketch "Sketch2 (2)" along normal blind 17 contours L1 L3 L4 L5 L6 L7 L8 bodies 11 in component "Geruesthalterung Top"
extrude "Extrude3'''" add sketch "Sketch1 (4)" against normal blind 5 from surface at 163 separate body contours L3 L4 L5 A3 A4 L6 L7 makes body 12 in component "Geruesthalterung Top"
extrude "Extrude4'''" add sketch "Sketch2 (2)" against normal blind 17 from surface at -163 contours L1 L3 L4 L5 L6 L7 L8 bodies 12 in component "Geruesthalterung Top"
sketch "Sketch3 (2)" plane through (0, 5.5, 0) normal (0, -1, 0) x (1, 0, 0) in component "Geruesthalterung Top"
  line L0 (1.5, 149.5) -> (1.5, 169.5)
  line L1 (1.5, 169.5) -> (-15.5, 169.5)
  line L2 (-15.5, 169.5) -> (-15.5, 149.5)
  line L3 (-15.5, 149.5) -> (1.5, 149.5)
  line L4 (1.5, 159.5) -> (-15.5, 159.5) construction
  line L5 (-7, 169.5) -> (-7, 149.5) construction
  circle A0 centre (-7, 159.5) radius 5.5
  circle A1 centre (-7, 159.5) radius 2.75
  dimension "d222" = 11
  dimension "d223" = 5.5
  constraint midpoint L0 L4.start
  constraint midpoint L2 L4.end
  constraint midpoint L1 L5.start
  constraint midpoint L3 L5.end
  constraint midpoint L5 A0.centre
  constraint concentric A0 A1
  measures "d222" diameter of A0
  measures "d223" diameter of A1
sketch "Sketch4 (4)" plane through (0, 5.5, 0) normal (0, -1, 0) x (1, 0, 0) in component "Geruesthalterung Top"
  line L0 (164.5, 169.5) -> (164.5, 149.5)
  line L1 (164.5, 149.5) -> (181.5, 149.5)
  line L2 (181.5, 149.5) -> (181.5, 169.5)
  line L3 (181.5, 169.5) -> (164.5, 169.5)
  line L4 (173, 169.5) -> (173, 149.5) construction
  line L5 (181.5, 159.5) -> (164.5, 159.5) construction
  circle A0 centre (173, 159.5) radius 5.5
  circle A1 centre (173, 159.5) radius 2.75
  dimension "d224" = 11
  dimension "d225" = 5.5
  constraint midpoint L3 L4.start
  constraint midpoint L1 L4.end
  constraint midpoint L2 L5.start
  constraint midpoint L0 L5.end
  constraint midpoint L5 A0.centre
  constraint concentric A0 A1
  measures "d224" diameter of A0
  measures "d225" diameter of A1
extrude "Extrude5''" cut sketch "Sketch4 (4)" sketch "Sketch3 (2)" along normal up to surface contours A1 of sketch 2 contours A1 end surface through (164.5, 10.5, 169.5) normal (0, 1, 0) offset 0 bodies 11 12 in component "Geruesthalterung Top"
extrude "Extrude6''" cut sketch "Sketch4 (4)" sketch "Sketch3 (2)" against normal blind 2 contours A0 of sketch 2 contours A0 bodies 11 12 in component "Geruesthalterung Top"
sketch "Sketch5 (3)" plane through (0, 10.5, 0) normal (0, 1, 0) x (-1, 0, 0) in component "Geruesthalterung Top"
  circle A0 centre (7, 159.5) radius 2.75
  line L0 (-6.5, 149.5) -> (15.5, 149.5)
  line L1 (15.5, 149.5) -> (15.5, 169.5)
  line L2 (15.5, 169.5) -> (-6.5, 169.5)
  line L3 (-6.5, 169.5) -> (-6.5, 149.5)
  line L4 (15.5, 159.5) -> (-6.5, 159.5) construction
  line L5 (-6.5, 162) -> (-4.5, 162)
  line L6 (-4.5, 162) -> (-4.5, 157)
  line L7 (-4.5, 157) -> (-6.5, 157)
  line L8 (-6.5, 157) -> (-6.5, 162)
  line L9 (-6.5, 162) -> (-4.5, 157) construction
  line L10 (-4.5, 162) -> (-6.5, 157) construction
  point P0 (-5.5, 159.5)
  dimension "d231" = 5
  dimension "d232" = 2
  constraint midpoint L1 L4.start
  constraint coincident L3 L4.end
  constraint perpendicular L3 L4
  constraint perpendicular L5 L6
  constraint parallel L5 L7
  constraint parallel L6 L8
  constraint horizontal L5
  constraint coincident L3 L5.start
  constraint coincident L9 P0
  constraint coincident L10 P0
  constraint coincident L4 P0
  measures "d231" distance of L5.start L7.end
  measures "d232" distance of L5.start L5.end
sketch "Sketch6 (2)" plane through (0, 10.5, 0) normal (0, 1, 0) x (-1, 0, 0) in component "Geruesthalterung Top"
  circle A0 centre (-173, 159.5) radius 2.75
  line L0 (-159.5, 149.5) -> (-159.5, 169.5)
  line L1 (-159.5, 169.5) -> (-181.5, 169.5)
  line L2 (-181.5, 169.5) -> (-181.5, 149.5)
  line L3 (-181.5, 149.5) -> (-159.5, 149.5)
  line L4 (-181.5, 159.5) -> (-159.5, 159.5) construction
  line L5 (-161.5, 162) -> (-159.5, 162)
  line L6 (-159.5, 162) -> (-159.5, 157)
  line L7 (-159.5, 157) -> (-161.5, 157)
  line L8 (-161.5, 157) -> (-161.5, 162)
  line L9 (-161.5, 162) -> (-159.5, 157) construction
  line L10 (-159.5, 162) -> (-161.5, 157) construction
  point P0 (-160.5, 159.5)
  dimension "d233" = 5
  dimension "d234" = 2
  constraint midpoint L2 L4.start
  constraint coincident L0 L4.end
  constraint perpendicular L0 L4
  constraint perpendicular L5 L6
  constraint parallel L5 L7
  constraint parallel L6 L8
  constraint horizontal L5
  constraint coincident L9 P0
  constraint coincident L10 P0
  constraint coincident L4 P0
  constraint collinear L0 L6
  measures "d233" distance of L5.end L6.end
  measures "d234" distance of L6.end L7.end
extrude "Extrude7''" add sketch "Sketch6 (2)" sketch "Sketch5 (3)" along normal blind 2 contours L0 L5 L6 L7 L8 of sketch 2 contours L3 L5 L6 L7 L8 bodies 11 12 in component "Geruesthalterung Top"
sketch "Sketch1 (5)" plane through (1.5, 0, 0) normal (1, 0, 0) x (0, 1, 0) in component "Geruesthalterung Bot"
  circle A0 centre (11.1258, -19.1055) radius 4.4
  circle A1 centre (32.0375, -14.9459) radius 4.4
  circle A2 centre (52.2274, -8.0924) radius 4.4
  circle A3 centre (71.35, 1.3379) radius 4.4
  circle A4 centre (105.1084, 27.2416) radius 4.4
  circle A5 centre (89.0781, 13.1834) radius 4.4
  circle A6 centre (-10.15, -20.5) radius 4.4 construction
  arc A7 (-10.15, -30.5) -> (112.1795, 20.1705) centre (-10.15, 142.5) ccw construction
  arc A8 (112.1795, 20.1705) -> (98.0373, 34.3127) centre (105.1084, 27.2416) ccw
  arc A9 (2.5, -9.9762) -> (98.0373, 34.3127) centre (-10.15, 142.5) ccw
  line L0 (2.5, -9.9762) -> (2.5, -3.5)
  line L1 (2.5, -3.5) -> (-22.8, -3.5)
  line L2 (-22.8, -3.5) -> (-22.8, -20.5)
  arc A10 (-22.8, -20.5) -> (-12.8, -30.5) centre (-12.8, -20.5) ccw construction
  line L3 (-12.8, -30.5) -> (-10.15, -30.5) construction
  circle A11 centre (-10.15, -20.5) radius 3.75
  line L4 (-10.15, -50.5) -> (7.85, -50.5)
  line L5 (-0.15, -30.5) -> (-0.15, -20.5)
  line L6 (-20.15, -20.5) -> (-20.15, -40.5)
  arc A12 (-0.15, -20.5) -> (-20.15, -20.5) centre (-10.15, -20.5) ccw
  arc A13 (-20.15, -40.5) -> (-10.15, -50.5) centre (-10.15, -40.5) ccw
  line L7 (7.85, -50.5) -> (7.85, -30.5)
  line L8 (7.85, -30.5) -> (-0.15, -30.5)
  dimension "d237" = 7.5
  dimension "d238" = 20
  dimension "d271" = 10
  dimension "d278" = 8
  dimension "d280" = 10
  dimension "d281" = 20
  constraint concentric A6 A11
  constraint concentric A11 A12
  constraint vertical L5
  constraint vertical L6
  constraint tangent L5 A12
  constraint tangent L6 A12
  constraint tangent L4 A13
  constraint tangent L6 A13
  constraint vertical L7
  constraint horizontal L8
  constraint horizontal L4
  measures "d237" diameter of A11
  measures "d238" diameter of A12
  measures "d271" radius of A13
  measures "d278" distance of L7.end L5.start
  measures "d280" distance of L5.end L5.start
  measures "d281" distance of L4 L8
extrude "Extrude1''''" add sketch "Sketch1 (5)" against normal blind 7 separate body contours A11 makes body 13 in component "Geruesthalterung Bot"
extrude "Extrude2''''" add sketch "Sketch1 (5)" along normal blind 5 contours A11 | L4 L5 L6 A12 A13 L7 L8 bodies 13 in component "Geruesthalterung Bot"
extrude "Extrude3''''" add sketch "Sketch1 (5)" along normal blind 7 from surface at 163 separate body contours A11 makes body 14 in component "Geruesthalterung Bot"
extrude "Extrude4''''" add sketch "Sketch1 (5)" against normal blind 5 from surface at 163 contours A11 | L4 L5 L6 A12 A13 L7 L8 bodies 14 in component "Geruesthalterung Bot"
sketch "Sketch2 (3)" plane through (1.5, 0, 0) normal (-1, 0, 0) x (0, -1, 0) in component "Geruesthalterung Bot"
  arc A0 (20.15, -20.5) -> (0.15, -20.5) centre (10.15, -20.5) ccw
  line L0 (0.15, -20.5) -> (0.15, -30.5)
  line L1 (-7.85, -50.5) -> (10.15, -50.5)
  line L2 (20.15, -40.5) -> (20.15, -20.5)
  circle A1 centre (10.15, -20.5) radius 3.75
  line L3 (-7.85, -50.5) -> (-2.85, -50.5)
  line L4 (-2.85, -50.5) -> (-2.85, -30.5)
  line L5 (-2.85, -30.5) -> (-7.85, -30.5)
  line L6 (-7.85, -30.5) -> (-7.85, -50.5)
  arc A2 (10.15, -50.5) -> (20.15, -40.5) centre (10.15, -40.5) ccw
  line L7 (0.15, -30.5) -> (-7.85, -30.5)
  line L8 (-7.85, -30.5) -> (-7.85, -50.5)
  dimension "d250" = 20
  dimension "d251" = 5
  constraint horizontal L3
  constraint vertical L4
  constraint horizontal L5
  constraint vertical L6
  constraint coincident L1.start L3.start
  measures "d250" distance of L1.start L5.end
  measures "d251" distance of L1.start L3.end
extrude "Extrude5'''" add sketch "Sketch2 (3)" along normal blind 17 contours L1 L3 L4 L5 L6 L7 L8 bodies 13 in component "Geruesthalterung Bot"
extrude "Extrude6'''" add sketch "Sketch2 (3)" against normal blind 17 from surface at -163 contours L1 L3 L4 L5 L6 L7 L8 bodies 14 in component "Geruesthalterung Bot"
sketch "Sketch3 (3)" plane through (0, 2.85, 0) normal (0, -1, 0) x (1, 0, 0) in component "Geruesthalterung Bot"
  line L0 (1.5, -50.5) -> (1.5, -30.5)
  line L1 (1.5, -30.5) -> (-15.5, -30.5)
  line L2 (-15.5, -30.5) -> (-15.5, -50.5)
  line L3 (-15.5, -50.5) -> (1.5, -50.5)
  line L4 (-15.5, -40.5) -> (1.5, -40.5) construction
  line L5 (-7, -30.5) -> (-7, -50.5) construction
  circle A0 centre (-7, -40.5) radius 5.5
  circle A1 centre (-7, -40.5) radius 2.75
  dimension "d257" = 11
  dimension "d258" = 5.5
  constraint midpoint L2 L4.start
  constraint midpoint L0 L4.end
  constraint midpoint L1 L5.start
  constraint midpoint L3 L5.end
  constraint midpoint L5 A0.centre
  constraint concentric A0 A1
  measures "d257" diameter of A0
  measures "d258" diameter of A1
sketch "Sketch4 (5)" plane through (0, 2.85, 0) normal (0, -1, 0) x (1, 0, 0) in component "Geruesthalterung Bot"
  line L0 (164.5, -30.5) -> (164.5, -50.5)
  line L1 (164.5, -50.5) -> (181.5, -50.5)
  line L2 (181.5, -50.5) -> (181.5, -30.5)
  line L3 (181.5, -30.5) -> (164.5, -30.5)
  line L4 (164.5, -40.5) -> (181.5, -40.5) construction
  line L5 (173, -30.5) -> (173, -50.5) construction
  circle A0 centre (173, -40.5) radius 5.5
  circle A1 centre (173, -40.5) radius 2.75
  dimension "d259" = 11
  dimension "d260" = 5.5
  constraint midpoint L0 L4.start
  constraint midpoint L2 L4.end
  constraint midpoint L3 L5.start
  constraint midpoint L1 L5.end
  constraint midpoint L4 A0.centre
  constraint concentric A0 A1
  measures "d259" diameter of A0
  measures "d260" diameter of A1
extrude "Extrude7'''" cut sketch "Sketch4 (5)" sketch "Sketch3 (3)" along normal up to surface contours A1 of sketch 2 contours A1 end surface through (164.5, 7.85, -30.5) normal (0, 1, 0) offset 0 bodies 13 14 in component "Geruesthalterung Bot"
extrude "Extrude8'" cut sketch "Sketch4 (5)" sketch "Sketch3 (3)" against normal blind 2 contours A0 of sketch 2 contours A0 bodies 13 14 in component "Geruesthalterung Bot"
sketch "Sketch5 (4)" plane through (0, 7.85, 0) normal (0, 1, 0) x (-1, 0, 0) in component "Geruesthalterung Bot"
  circle A0 centre (7, -40.5) radius 2.75
  line L0 (-6.5, -30.5) -> (-6.5, -50.5)
  line L1 (-6.5, -50.5) -> (15.5, -50.5)
  line L2 (15.5, -50.5) -> (15.5, -30.5)
  line L3 (15.5, -30.5) -> (-6.5, -30.5)
  line L4 (15.5, -40.5) -> (-6.5, -40.5) construction
  line L5 (-6.5, -38) -> (-4.5, -38)
  line L6 (-4.5, -38) -> (-4.5, -43)
  line L7 (-4.5, -43) -> (-6.5, -43)
  line L8 (-6.5, -43) -> (-6.5, -38)
  line L9 (-6.5, -38) -> (-4.5, -43) construction
  line L10 (-4.5, -38) -> (-6.5, -43) construction
  point P0 (-5.5, -40.5)
  dimension "d265" = 5
  dimension "d266" = 2
  constraint midpoint L2 L4.start
  constraint coincident L0 L4.end
  constraint perpendicular L0 L4
  constraint perpendicular L5 L6
  constraint parallel L5 L7
  constraint parallel L6 L8
  constraint horizontal L5
  constraint coincident L9 P0
  constraint coincident L10 P0
  constraint coincident L4 P0
  constraint collinear L0 L8
  measures "d265" distance of L5.end L6.end
  measures "d266" distance of L6.end L7.end
sketch "Sketch6 (3)" plane through (0, 7.85, 0) normal (0, 1, 0) x (-1, 0, 0) in component "Geruesthalterung Bot"
  circle A0 centre (-173, -40.5) radius 2.75
  line L0 (-181.5, -50.5) -> (-159.5, -50.5)
  line L1 (-159.5, -50.5) -> (-159.5, -30.5)
  line L2 (-159.5, -30.5) -> (-181.5, -30.5)
  line L3 (-181.5, -30.5) -> (-181.5, -50.5)
  line L4 (-181.5, -40.5) -> (-159.5, -40.5) construction
  line L5 (-159.5, -38) -> (-161.5, -38)
  line L6 (-161.5, -38) -> (-161.5, -43)
  line L7 (-161.5, -43) -> (-159.5, -43)
  line L8 (-159.5, -43) -> (-159.5, -38)
  line L9 (-159.5, -38) -> (-161.5, -43) construction
  line L10 (-161.5, -38) -> (-159.5, -43) construction
  point P0 (-160.5, -40.5)
  dimension "d267" = 5
  dimension "d268" = 2
  constraint midpoint L3 L4.start
  constraint coincident L1 L4.end
  constraint perpendicular L1 L4
  constraint perpendicular L5 L6
  constraint parallel L5 L7
  constraint parallel L6 L8
  constraint horizontal L5
  constraint coincident L9 P0
  constraint coincident L10 P0
  constraint coincident L4 P0
  constraint collinear L1 L8
  measures "d267" distance of L5.end L6.end
  measures "d268" distance of L6.end L7.end
extrude "Extrude9'" add sketch "Sketch5 (4)" sketch "Sketch6 (3)" along normal blind 2 contours L0 L5 L6 L7 L8 of sketch 2 contours L1 L5 L6 L7 L8 bodies 13 14 in component "Geruesthalterung Bot"
component "Frame" placed x (1, 0, 0) y (0, 1, 0) z (0, 0, 1) at (0, 0, 0)
component "Abdeckung Hinten" placed x (1, 0, 0) y (0, 1, 0) z (0, 0, 1) at (0, 0, 0)
component "Display Halterung" placed x (1, 0, 0) y (0, 1, 0) z (0, 0, 1) at (0, 0, 0)
component "Geruesthalterung Top" placed x (1, 0, 0) y (0, 1, 0) z (0, 0, 1) at (0, 0, 0)
component "Geruesthalterung Bot" placed x (1, 0, 0) y (0, 1, 0) z (0, 0, 1) at (0, 0, 0)
equation "d3 = d2"
equation "d6 = d2"
equation "d7 = d2"
equation "d12 = d11"
equation "d15 = d2"
equation "d16 = d2"
equation "d17 = d2"
equation "d18 = d2"
equation "d19 = d2"
equation "d20 = d2"
equation "d21 = d2"
equation "d22 = d2"
equation "d23 = d2"
equation "d24 = d2"
equation "d26 = d2"
equation "d27 = d2"
equation "d28 = d2"
equation "d30 = d29"
equation "d45 = d44"
equation "d48 = d47"
equation "d51 = d50"
equation "d82 = d81"
equation "d83 = d81"
equation "d84 = d81"
equation "d128 = d127"
equation "d129 = d127"
equation "d130 = d127"
equation "d200 = 25.30 mm / 2"
